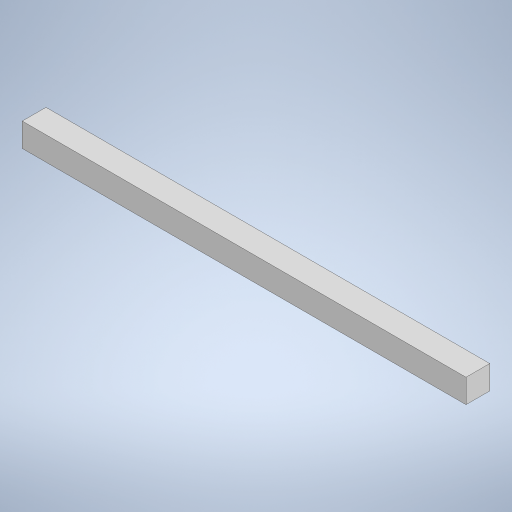
# Autodesk Inventor part: BarraHorizontal
Saved by Autodesk Inventor 2024 (Build 280153000, 153)
## iProperties
Created: 2023-06-28
Part Number: BarraHorizontal
Material: Genérico
Document SubType Name: Modeling
Designer: Personal
Density: 1 g/cm^3
Appearance: Valor por defecto
Author: Personal
Autodesk Inventor part; units mm, degrees
ref_plane "YZ Plane" through (0, 0, 0) normal (1, 0, 0) x (0, 1, 0)
ref_plane "XZ Plane" through (0, 0, 0) normal (0, 1, 0) x (-1, 0, 0)
ref_plane "XY Plane" through (0, 0, 0) normal (0, 0, 1) x (1, 0, 0)
sketch "Boceto1" plane through (0, 0, 0) normal (0, 0, 1) x (1, 0, 0)
  line L0 (9, 0) -> (9, 207.6) construction
  line L1 (0, 0) -> (0, 207.6) construction
  line L2 (0, 207.6) -> (-168.2, 207.6)
  line L3 (-168.2, 207.6) -> (-168.2, 198.6)
  line L4 (-168.2, 198.6) -> (0, 198.6)
  line L5 (0, 198.6) -> (0, 207.6)
  dimension "d0" = 9
  dimension "d3" = 168.2
  constraints: 8 end point, 2 parallel, 1 horizontal, 1 perpendicular
  measures "d0" distance between parallel lines of L4 L2
  measures "d3" distance of L1.end L2.end
extrude "Extrusión1" add sketch "Boceto1" along normal blind 9
